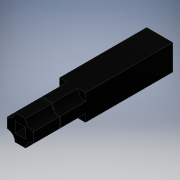
# Autodesk Inventor part: SMT GPIO Female Header 2x20
Saved by Autodesk Inventor 2016 (Build 200138000, 138)
## iProperties
Created: 2016-07-25
Part Number: SMT GPIO Female Header 2x20
Material: Generic
Document SubType Name: Modeling
Designer: Jonathan
Density: 1 g/cm^3
Appearance: Smooth - Black
Author: Jonathan
Autodesk Inventor part; units mm, degrees
ref_plane "YZ Plane" through (0, 0, 0) normal (1, 0, 0) x (0, 1, 0)
ref_plane "XZ Plane" through (0, 0, 0) normal (0, 1, 0) x (-1, 0, 0)
ref_plane "XY Plane" through (0, 0, 0) normal (0, 0, 1) x (1, 0, 0)
sketch "Sketch1" plane through (0, 0, 0) normal (0, 1, 0) x (-1, 0, 0)
  line L0 (1.27, 1.25) -> (-1.27, 1.25)
  line L1 (-1.27, 1.25) -> (-1.27, -1.25)
  line L2 (-1.27, -1.25) -> (1.27, -1.25)
  line L3 (1.27, -1.25) -> (1.27, 1.25)
  line L4 (1.27, 1.25) -> (-1.27, -1.25) construction
  line L5 (-1.27, 1.25) -> (1.27, -1.25) construction
  point P0 (0, 0)
  dimension "d0" = 2.54
  dimension "d1" = 2.5
  constraints: 12 end point, 2 midpoint, 2 parallel, 1 horizontal, 1 perpendicular
  measures "d0" distance of L1.end L2.end
  measures "d1" distance of L0.end L1.end
extrude "Extrusion1" add sketch "Sketch1" along normal blind 8.5
sketch "Sketch2" plane through (0, 0, 0) normal (0, -1, 0) x (1, 0, 0)
  line L0 (-1.27, 1.25) -> (1.27, 1.25) projected
  arc A0 (0.52, 1.25) -> (1.27, 0.5) centre (1.27, 1.25) ccw
  line L1 (-1.27, -1.25) -> (-1.27, 1.25) projected
  arc A1 (-1.27, 0.5) -> (-0.52, 1.25) centre (-1.27, 1.25) ccw
  arc A2 (-0.52, -1.25) -> (-1.27, -0.5) centre (-1.27, -1.25) ccw
  line L2 (1.27, -1.25) -> (-1.27, -1.25) projected
  arc A3 (1.27, -0.5) -> (0.52, -1.25) centre (1.27, -1.25) ccw
  line L3 (1.27, 1.25) -> (1.27, -1.25) projected
  line L4 (-1.27, -1.25) -> (-1.27, 1.25) projected
  line L5 (1.27, -1.25) -> (-1.27, -1.25) projected
  point P0 (0, 0)
  dimension "d4" = 0.75
  constraints: 8 point on circle, 8 point on line, 4 centre point, 4 coincident, 3 equal radius
  measures "d4" radius of A1
extrude "Extrusion2" add sketch "Sketch2" along normal blind 2.4 contours L0 A0 L3 A3 L2 A2 L1 A1
sketch "Sketch3" plane through (0, -2.4, 0) normal (0, -1, 0) x (1, 0, 0)
  line L0 (-1.125, 1.125) -> (1.125, 1.125)
  line L1 (1.125, 1.125) -> (1.125, -1.125)
  line L2 (1.125, -1.125) -> (-1.125, -1.125)
  line L3 (-1.125, -1.125) -> (-1.125, 1.125)
  line L4 (-1.125, 1.125) -> (1.125, -1.125) construction
  line L5 (1.125, 1.125) -> (-1.125, -1.125) construction
  arc A0 (-1.125, 0.3618) -> (-0.3787, 1.125) centre (-1.27, 1.25) ccw
  arc A1 (0.3787, 1.125) -> (1.125, 0.3618) centre (1.27, 1.25) ccw
  arc A2 (-0.3787, -1.125) -> (-1.125, -0.3618) centre (-1.27, -1.25) ccw
  arc A3 (1.125, -0.3618) -> (0.3787, -1.125) centre (1.27, -1.25) ccw
  point P0 (0, 0)
  dimension "d7" = 2.25
  dimension "d8" = 0.9
  dimension "d9" = 0.9
  dimension "d10" = 0.9
  dimension "d11" = 0.9
  constraints: 12 end point, 8 point on circle, 8 point on line, 4 centre point, 4 coincident, 2 midpoint, 2 parallel, 2 perpendicular, 1 horizontal
  measures "d7" distance of L0.start L0.end
  measures "d8" radius of A0
  measures "d9" radius of A1
  measures "d10" radius of A3
  measures "d11" radius of A2
extrude "Extrusion3" add sketch "Sketch3" along normal blind 0.14 contours L0 A1 L1 A3 L2 A2 L3 A0
sketch "Sketch4" plane through (0, -2.54, 0) normal (0, -1, 0) x (1, 0, 0)
  line L0 (0.52, 1.25) -> (-0.52, 1.25) projected
  arc A0 (-1.27, 0.5) -> (-0.52, 1.25) centre (-1.27, 1.25) ccw projected
  line L1 (-1.27, 0.5) -> (-1.27, -0.5) projected
  arc A1 (-0.52, -1.25) -> (-1.27, -0.5) centre (-1.27, -1.25) ccw projected
  line L2 (-0.52, -1.25) -> (0.52, -1.25) projected
  arc A2 (1.27, -0.5) -> (0.52, -1.25) centre (1.27, -1.25) ccw projected
  line L3 (1.27, -0.5) -> (1.27, 0.5) projected
  arc A3 (0.52, 1.25) -> (1.27, 0.5) centre (1.27, 1.25) ccw projected
  point P0 (0, 0)
extrude "Extrusion4" add sketch "Sketch4" along normal blind 2.54
sketch "Sketch5" plane through (0, 8.5, 0) normal (0, 1, 0) x (1, 0, 0)
  line L0 (-0.5, 0.5) -> (0.5, 0.5)
  line L1 (0.5, 0.5) -> (0.5, -0.5)
  line L2 (0.5, -0.5) -> (-0.5, -0.5)
  line L3 (-0.5, -0.5) -> (-0.5, 0.5)
  line L4 (-0.5, 0.5) -> (0.5, -0.5) construction
  line L5 (0.5, 0.5) -> (-0.5, -0.5) construction
  point P0 (0, 0)
  dimension "d16" = 1
  constraints: 12 end point, 2 midpoint, 2 parallel, 2 perpendicular, 1 horizontal
  measures "d16" distance of L0.start L0.end
extrude "Extrusion5" cut sketch "Sketch5" against normal through all
chamfer "Chamfer1" distance 0.5 angle 45 4 edges at (0, 8.5, -0.5) (-0.5, 8.5, 0) (0, 8.5, 0.5) (0.5, 8.5, 0)
body "Solid1"
